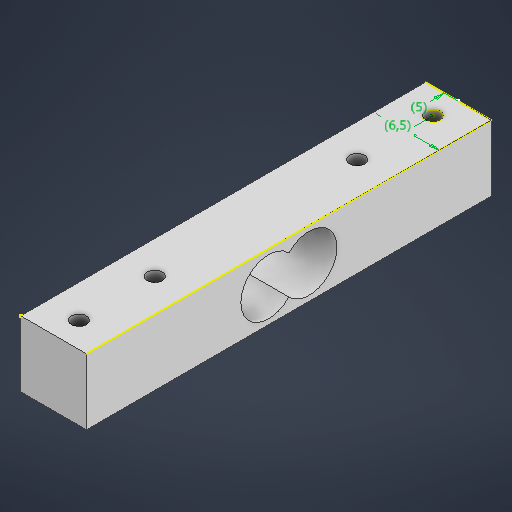
# Autodesk Inventor part: cella di carico
Saved by Autodesk Inventor 2026.2 (Build 302298000, 298)
## iProperties
Created: 2026-01-19
Part Number: cella di carico
Material: Generic
Document SubType Name: Modeling
Designer: ASUS
Density: 1 g/cm^3
Appearance: Default
Author: ASUS
Autodesk Inventor part; units mm, degrees
ref_plane "YZ Plane" through (0, 0, 0) normal (1, 0, 0) x (0, 1, 0)
ref_plane "XZ Plane" through (0, 0, 0) normal (0, 1, 0) x (-1, 0, 0)
ref_plane "XY Plane" through (0, 0, 0) normal (0, 0, 1) x (1, 0, 0)
sketch "Sketch1" plane through (0, 0, 0) normal (0, 1, 0) x (-1, 0, 0)
  line L0 (0, 0) -> (-13, 0)
  line L1 (0, 0) -> (-13, 0)
  line L2 (-13, 0) -> (-13, -80)
  line L3 (-13, -80) -> (0, -80)
  line L4 (0, -80) -> (0, 0)
  circle A0 centre (-6.5, -5) radius 1.5
  circle A1 centre (-6.5, -20) radius 1.5
  circle A2 centre (-6.5, -75) radius 1.5
  circle A3 centre (-6.5, -60) radius 1.5
  dimension "d1" = 13
  dimension "d2" = 80
  dimension "d4" = 3
  dimension "d6" = 3
  constraints: 10 end point, 4 centre point, 2 horizontal, 2 parallel, 1 perpendicular
  measures "d1" distance of L3.end L2.end
  measures "d2" distance of L2.end L1.end
  measures "d4" diameter of A0
  measures "d6" diameter of A1
extrude "Extrusion1" add sketch "Sketch1" along normal blind 13
sketch "Sketch2" plane through (13, 0, 0) normal (1, 0, 0) x (0, 0, -1)
  line L0 (0, 13) -> (80, 13) projected
  line L1 (40, 13) -> (40, 0)
  line L2 (0, 0) -> (80, 0) projected
  arc A0 (40, 10.2749) -> (40, 2.7251) centre (36, 6.5) ccw
  arc A1 (40, 2.7251) -> (40, 10.2749) centre (44, 6.5) ccw
  dimension "d10" = 11
  constraints: 4 point on circle, 2 centre point, 2 end point, 2 midpoint, 1 symmetric about line, 1 other
  measures "d10" diameter of A0
extrude "Extrusion2" cut sketch "Sketch2" against normal blind 13
sketch "Sketch3" plane through (0, 13, 0) normal (0, 1, 0) x (1, 0, 0)
  line L0 (13, 80) -> (0, 80) projected
  circle A0 centre (6.5, 75) radius 1.5 projected
  line L1 (13, 0) -> (13, 80) projected
  point P0 (0, 0)
  point P1 (6.5, 80)
  dimension "d13" = 5
  dimension "d14" = 6.5
  constraints: 1 midpoint
  measures "d13" distance of point (6.5, 80) A0.centre
  measures "d14" distance from line of L1 A0.centre
body "Solid1"
